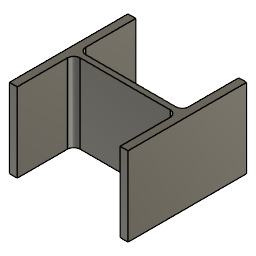
H-150×150×7×10 (Autodesk Fusion 360 design; units mm, degrees)
Autodesk Fusion 360 part; units mm, degrees
sketch "スケッチ1" plane through (0, 0, 0) normal (0, 0, 1) x (1, 0, 0)
  line L0 (0, 75) -> (0, -75)
  line L1 (150, -75) -> (150, 75)
  line L2 (140, -11.5) -> (140, -75)
  line L3 (10, -75) -> (10, -11.5)
  line L4 (0, -75) -> (10, -75)
  line L5 (140, -75) -> (150, -75)
  line L6 (10, 11.5) -> (10, 75)
  line L7 (140, 75) -> (140, 11.5)
  line L8 (18, -3.5) -> (132, -3.5)
  line L9 (132, 3.5) -> (18, 3.5)
  line L10 (10, 75) -> (0, 75)
  line L11 (150, 75) -> (140, 75)
  arc A0 (18, -3.5) -> (10, -11.5) centre (18, -11.5) ccw
  arc A1 (10, 11.5) -> (18, 3.5) centre (18, 11.5) ccw
  arc A2 (132, 3.5) -> (140, 11.5) centre (132, 11.5) ccw
  arc A3 (140, -11.5) -> (132, -3.5) centre (132, -11.5) ccw
extrude "押し出し1" add sketch "スケッチ1" along normal blind 100
